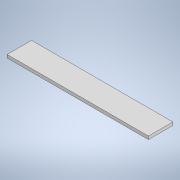
# Autodesk Inventor part: topForKetchenLight
Saved by Autodesk Inventor 2021.2 (Build 252289000, 289)
## iProperties
Created: 2021-02-17
Part Number: topForKetchenLight
Material: Generic
Document SubType Name: Modeling
Designer: robst
Density: 1 g/cm^3
Appearance: Default
Author: robst
Autodesk Inventor part; units mm, degrees
ref_plane "YZ Plane" through (0, 0, 0) normal (1, 0, 0) x (0, 1, 0)
ref_plane "XZ Plane" through (0, 0, 0) normal (0, 1, 0) x (-1, 0, 0)
ref_plane "XY Plane" through (0, 0, 0) normal (0, 0, 1) x (1, 0, 0)
sketch "Sketch2" plane through (0, 0, 0) normal (0, 1, 0) x (-1, 0, 0)
  line L0 (142.875, 24.6767) -> (-142.875, 24.6767)
  line L1 (-142.875, 24.6767) -> (-142.875, -24.6767)
  line L2 (-142.875, -24.6767) -> (142.875, -24.6767)
  line L3 (142.875, -24.6767) -> (142.875, 24.6767)
  line L4 (142.875, 24.6767) -> (-142.875, -24.6767) construction
  line L5 (-142.875, 24.6767) -> (142.875, -24.6767) construction
  point P0 (0, 0)
  dimension "d0" = 49.3535
  dimension "d1" = 285.75
  constraints: 12 end point, 2 midpoint, 2 parallel, 1 horizontal, 1 perpendicular
  measures "d0" distance of L2.end L0.start
  measures "d1" distance of L1.end L2.end
extrude "Extrusion1" add sketch "Sketch2" along normal blind 6.35
equation "\"d0\" = depth"
equation "\"d1\" = width"
equation "\"d2\" = thickness"
equation "\"width\" = 285.75"
equation "\"depth\" = 49.35347"
equation "\"thickness\" = 6.35"
body "Solid1"
